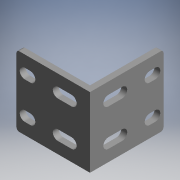
# Autodesk Inventor part: HPTBDW5-SEP_b.
Saved by Autodesk Inventor 2017.3 (Build 213256000, 256)
## iProperties
Part Number: HPTBDW5-SEP_b.
Material: Generic
Catalog Web Link: www.cadenas.de
Description: HPTBS5, SHPTBS5, HPTBD5, SHPTBD5, HPTBDW5, SHPTBDW5, HPTGS5_body-Sheet Metal Brackets - For HFS5 Series - Bent Type
Vendor: MISUMI
Document SubType Name: Modeling
Designer: partserver
Manufacturer: MISUMI
Mass: 7.98529 g
Surface Area: 64.2842 cm^2
Volume: 7.98529 cm^3
Density: 1 g/cm^3
Appearance: PSOLRGB-175-175-175
Category: PARTsolutions
Company: MISUMI
Title: HPTBDW5-SEP
Author: Cadenas PARTsolutions
Comments: Sheet Metal Brackets - For HFS5 Series - Bent Type
PSOL_IDENT_0: {$CADENAS_DATA\23d-libs\misumi\metric\38_al_extrusions_blackets\5\hptbs5\hptbs5.prj},241 {VTYP=3D},{
PSOL_IDENT_1: NB=HPTBDW5-SEP_b.},{LINA=HPTBDW5-SEP},{NN=HPTBS5, SHPTBS5, HPTBD5, SHPTBD5, HPTBDW5, SHPTBDW5, HPTGS
PSOL_IDENT_2: 5_body},{DATE=08.06.2021 08:25:19},{GEOMDATE=24.03.2020 04:31:18},{VERSION=},{LINEID=270},{WBVAR=MAT
PSOL_IDENT_3: ,SHPT,NOH,ALT1},{WBNUMERIC=}  {NB=HPTBDW5-SEP_b.},{LINA=HPTBDW5-SEP},{KT=5},{PN=HPTBDW5-SEP},{TYPE=H
PSOL_IDENT_4: PTBDW},{NO=5},{MAT=},{ST=Bright Chromate},{SHPT=L},{SHPTALG= 'L', 'L-Shaped Bent','B', 'Both Ends Be
PSOL_IDENT_5: mt' },{NOH=BDW},{NOHALG= 'BS','2','BD','4','BDW','8' },{MASS=58},{A=38},{B=40},{T=3.2},{N=5.5},{E=0.
PSOL_IDENT_6: 0},{W=20},{H=10.0},{G=7.5},{F=15},{R=1.5},{ALT1=-SEP},{AB=CBM5-8},{ABD=5},{ABL=8},{NOB=8},{AN=HNTP5-
PSOL_IDENT_7: 5},{NON=8},{AB1=5-8},{AN1=5-5},{MAT1='', 'Low Carbon Steel', 'S', '304 Stainless Steel'},{NUTMAT=101
PSOL_IDENT_8: 0 Carbon Steel Equivalent},{NUTTHREAD=5},{NUT1=5},{C=3.000}
NB: HPTBDW5-SEP_b.
NN: HPTBS5, SHPTBS5, HPTBD5, SHPTBD5, HPTBDW5, SHPTBDW5, HPTGS5_body
NT: Sheet Metal Brackets - For HFS5 Series - Bent Type
NBSYN: $PN._b.
LINA: HPTBDW5-SEP
CATALOG: Misumi
PN: HPTBDW5-SEP
NO: 5
MAT: Low Carbon Steel
ST: Bright Chromate
SHPT: L-Shaped Bent
NOH: 8
MASS: 58
T: 3.2
ALT1: with SEP (Post-Assembly Fitting Spring Nuts Set of Applicable Bolt and Nut)
AB: CBM5-8
NOB: 8
AN: HNTP5-5
NON: 8
SUPPLIER: MISUMI
ARTICLENO: HPTBDW5-SEP_b.
BOMINFO: HPTBDW5-SEP
CREATOR: CADENAS GmbH
Autodesk Inventor part; units mm, degrees
sketch "Sketch_1" plane through (0, 0, 0) normal (1, 0, 0) x (0, 1, 0)
  line L0 (38.5, 19) -> (0, 19)
  line L1 (0, 19) -> (0, -19)
  line L2 (0, -19) -> (38.5, -19)
  arc A0 (38.5, -19) -> (40, -17.5) centre (38.5, -17.5) ccw
  line L3 (40, -17.5) -> (40, 17.5)
  arc A1 (40, 17.5) -> (38.5, 19) centre (38.5, 17.5) ccw
  line L4 (17.5, -7.25) -> (10, -7.25)
  arc A2 (10, -7.25) -> (10, -12.75) centre (10, -10) ccw
  line L5 (10, -12.75) -> (17.5, -12.75)
  arc A3 (17.5, -12.75) -> (17.5, -7.25) centre (17.5, -10) ccw
  line L6 (35.5, -7.25) -> (32.5, -7.25)
  arc A4 (32.5, -7.25) -> (32.5, -12.75) centre (32.5, -10) ccw
  line L7 (32.5, -12.75) -> (35.5, -12.75)
  arc A5 (35.5, -12.75) -> (35.5, -7.25) centre (35.5, -10) ccw
  line L8 (17.5, 12.75) -> (10, 12.75)
  arc A6 (10, 12.75) -> (10, 7.25) centre (10, 10) ccw
  line L9 (10, 7.25) -> (17.5, 7.25)
  arc A7 (17.5, 7.25) -> (17.5, 12.75) centre (17.5, 10) ccw
  line L10 (35.5, 12.75) -> (32.5, 12.75)
  arc A8 (32.5, 12.75) -> (32.5, 7.25) centre (32.5, 10) ccw
  line L11 (32.5, 7.25) -> (35.5, 7.25)
  arc A9 (35.5, 7.25) -> (35.5, 12.75) centre (35.5, 10) ccw
  constraints: 24 end point, 20 point on circle, 10 centre point
extrude "Extrusion1" add sketch "Sketch_1" along normal blind 3.2
sketch "Sketch_3" plane through (0, 0, 0) normal (0, 1, 0) x (-1, 0, 0)
  line L0 (0, 19) -> (-38.5, 19)
  arc A0 (-38.5, 19) -> (-40, 17.5) centre (-38.5, 17.5) ccw
  line L1 (-40, 17.5) -> (-40, -17.5)
  arc A1 (-40, -17.5) -> (-38.5, -19) centre (-38.5, -17.5) ccw
  line L2 (-38.5, -19) -> (0, -19)
  line L3 (0, -19) -> (0, 19)
  arc A2 (-32.5, -12.75) -> (-32.5, -7.25) centre (-32.5, -10) ccw
  line L4 (-32.5, -7.25) -> (-35.5, -7.25)
  arc A3 (-35.5, -7.25) -> (-35.5, -12.75) centre (-35.5, -10) ccw
  line L5 (-35.5, -12.75) -> (-32.5, -12.75)
  arc A4 (-32.5, 7.25) -> (-32.5, 12.75) centre (-32.5, 10) ccw
  line L6 (-32.5, 12.75) -> (-35.5, 12.75)
  arc A5 (-35.5, 12.75) -> (-35.5, 7.25) centre (-35.5, 10) ccw
  line L7 (-35.5, 7.25) -> (-32.5, 7.25)
  arc A6 (-10, -12.75) -> (-10, -7.25) centre (-10, -10) ccw
  line L8 (-10, -7.25) -> (-17.5, -7.25)
  arc A7 (-17.5, -7.25) -> (-17.5, -12.75) centre (-17.5, -10) ccw
  line L9 (-17.5, -12.75) -> (-10, -12.75)
  arc A8 (-10, 7.25) -> (-10, 12.75) centre (-10, 10) ccw
  line L10 (-10, 12.75) -> (-17.5, 12.75)
  arc A9 (-17.5, 12.75) -> (-17.5, 7.25) centre (-17.5, 10) ccw
  line L11 (-17.5, 7.25) -> (-10, 7.25)
  constraints: 24 end point, 20 point on circle, 10 centre point
extrude "Extrusion2" add sketch "Sketch_3" along normal blind 3.2
ref_plane "to_cbm_1_1_XY" through (3.2, 17.5, -10) normal (1, 0, 0) x (0, 0, -1)
ref_plane "to_cbm_1_1_YZ" through (3.2, 17.5, -10) normal (0, 0, -1) x (0, 1, 0)
ref_plane "to_cbm_1_1_ZX" through (3.2, 17.5, -10) normal (0, 1, 0) x (1, 0, 0)
ref_plane "to_cbm_1_2_XY" through (3.2, 17.5, 10) normal (1, 0, 0) x (0, 0, -1)
ref_plane "to_cbm_1_2_YZ" through (3.2, 17.5, 10) normal (0, 0, -1) x (0, 1, 0)
ref_plane "to_cbm_1_2_ZX" through (3.2, 17.5, 10) normal (0, 1, 0) x (1, 0, 0)
ref_plane "to_cbm_1_3_XY" through (3.2, 35.5, -10) normal (1, 0, 0) x (0, 0, -1)
ref_plane "to_cbm_1_3_YZ" through (3.2, 35.5, -10) normal (0, 0, -1) x (0, 1, 0)
ref_plane "to_cbm_1_3_ZX" through (3.2, 35.5, -10) normal (0, 1, 0) x (1, 0, 0)
ref_plane "to_cbm_1_4_XY" through (3.2, 35.5, 10) normal (1, 0, 0) x (0, 0, -1)
ref_plane "to_cbm_1_4_YZ" through (3.2, 35.5, 10) normal (0, 0, -1) x (0, 1, 0)
ref_plane "to_cbm_1_4_ZX" through (3.2, 35.5, 10) normal (0, 1, 0) x (1, 0, 0)
ref_plane "to_cbm_2_1_XY" through (17.5, 3.2, 10) normal (0, 1, 0) x (1, 0, 0)
ref_plane "to_cbm_2_1_YZ" through (17.5, 3.2, 10) normal (1, 0, 0) x (0, 0, -1)
ref_plane "to_cbm_2_1_ZX" through (17.5, 3.2, 10) normal (0, 0, -1) x (0, 1, 0)
ref_plane "to_cbm_2_2_XY" through (17.5, 3.2, -10) normal (0, 1, 0) x (1, 0, 0)
ref_plane "to_cbm_2_2_YZ" through (17.5, 3.2, -10) normal (1, 0, 0) x (0, 0, -1)
ref_plane "to_cbm_2_2_ZX" through (17.5, 3.2, -10) normal (0, 0, -1) x (0, 1, 0)
ref_plane "to_cbm_2_3_XY" through (35.5, 3.2, 10) normal (0, 1, 0) x (1, 0, 0)
ref_plane "to_cbm_2_3_YZ" through (35.5, 3.2, 10) normal (1, 0, 0) x (0, 0, -1)
ref_plane "to_cbm_2_3_ZX" through (35.5, 3.2, 10) normal (0, 0, -1) x (0, 1, 0)
ref_plane "to_cbm_2_4_XY" through (35.5, 3.2, -10) normal (0, 1, 0) x (1, 0, 0)
ref_plane "to_cbm_2_4_YZ" through (35.5, 3.2, -10) normal (1, 0, 0) x (0, 0, -1)
ref_plane "to_cbm_2_4_ZX" through (35.5, 3.2, -10) normal (0, 0, -1) x (0, 1, 0)
ref_plane "to_hntp5_1_1_XY" through (-2, 17.5, -10) normal (-1, 0, 0) x (0, -1, 0)
ref_plane "to_hntp5_1_1_YZ" through (-2, 17.5, -10) normal (0, -1, 0) x (0, 0, 1)
ref_plane "to_hntp5_1_1_ZX" through (-2, 17.5, -10) normal (0, 0, 1) x (-1, 0, 0)
ref_plane "to_hntp5_1_2_XY" through (-2, 17.5, 10) normal (-1, 0, 0) x (0, -1, 0)
ref_plane "to_hntp5_1_2_YZ" through (-2, 17.5, 10) normal (0, -1, 0) x (0, 0, 1)
ref_plane "to_hntp5_1_2_ZX" through (-2, 17.5, 10) normal (0, 0, 1) x (-1, 0, 0)
ref_plane "to_hntp5_1_3_XY" through (-2, 35.5, -10) normal (-1, 0, 0) x (0, -1, 0)
ref_plane "to_hntp5_1_3_YZ" through (-2, 35.5, -10) normal (0, -1, 0) x (0, 0, 1)
ref_plane "to_hntp5_1_3_ZX" through (-2, 35.5, -10) normal (0, 0, 1) x (-1, 0, 0)
ref_plane "to_hntp5_1_4_XY" through (-2, 35.5, 10) normal (-1, 0, 0) x (0, -1, 0)
ref_plane "to_hntp5_1_4_YZ" through (-2, 35.5, 10) normal (0, -1, 0) x (0, 0, 1)
ref_plane "to_hntp5_1_4_ZX" through (-2, 35.5, 10) normal (0, 0, 1) x (-1, 0, 0)
ref_plane "to_hntp5_2_1_XY" through (17.5, -2, 10) normal (0, -1, 0) x (-1, 0, 0)
ref_plane "to_hntp5_2_1_YZ" through (17.5, -2, 10) normal (-1, 0, 0) x (0, 0, -1)
ref_plane "to_hntp5_2_1_ZX" through (17.5, -2, 10) normal (0, 0, -1) x (0, -1, 0)
ref_plane "to_hntp5_2_2_XY" through (17.5, -2, -10) normal (0, -1, 0) x (-1, 0, 0)
ref_plane "to_hntp5_2_2_YZ" through (17.5, -2, -10) normal (-1, 0, 0) x (0, 0, -1)
ref_plane "to_hntp5_2_2_ZX" through (17.5, -2, -10) normal (0, 0, -1) x (0, -1, 0)
ref_plane "to_hntp5_2_3_XY" through (35.5, -2, 10) normal (0, -1, 0) x (-1, 0, 0)
ref_plane "to_hntp5_2_3_YZ" through (35.5, -2, 10) normal (-1, 0, 0) x (0, 0, -1)
ref_plane "to_hntp5_2_3_ZX" through (35.5, -2, 10) normal (0, 0, -1) x (0, -1, 0)
ref_plane "to_hntp5_2_4_XY" through (35.5, -2, -10) normal (0, -1, 0) x (-1, 0, 0)
ref_plane "to_hntp5_2_4_YZ" through (35.5, -2, -10) normal (-1, 0, 0) x (0, 0, -1)
ref_plane "to_hntp5_2_4_ZX" through (35.5, -2, -10) normal (0, 0, -1) x (0, -1, 0)
body "Solid1"
